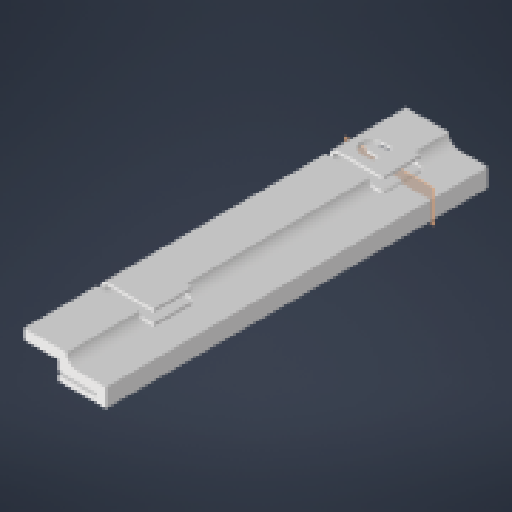
# Autodesk Inventor part: Tourniquet_Rail_01
Saved by Autodesk Inventor 2026.2 (Build 302298000, 298)
## iProperties
Created: 2026-03-04
Part Number: Tourniquet_Rail_01
Material: Generic
Document SubType Name: Modeling
Designer: vckot
Density: 1 g/cm^3
Appearance: Default
Author: vckot
Autodesk Inventor part; units mm, degrees
ref_plane "YZ Plane" through (0, 0, 0) normal (1, 0, 0) x (0, 1, 0)
ref_plane "XZ Plane" through (0, 0, 0) normal (0, 1, 0) x (-1, 0, 0)
ref_plane "XY Plane" through (0, 0, 0) normal (0, 0, 1) x (1, 0, 0)
sketch "Sketch1" plane through (0, 0, 0) normal (0, 1, 0) x (-1, 0, 0)
  line L0 (-6.25, 50) -> (6.25, 50)
  line L1 (6.25, 50) -> (6.25, -50)
  line L2 (6.25, -50) -> (-6.25, -50)
  line L3 (-6.25, -50) -> (-6.25, 50)
  line L4 (-6.25, 50) -> (6.25, -50) construction
  line L5 (6.25, 50) -> (-6.25, -50) construction
  point P0 (0, 0)
  dimension "d0" = 12.5
  dimension "d1" = 100
  constraints: 12 end point, 2 midpoint, 2 parallel, 1 horizontal, 1 perpendicular
  measures "d0" distance of L1.end L2.end
  measures "d1" distance of L0.end L1.end
extrude "Extrusion1" add sketch "Sketch1" along normal blind 4.8
sketch "Sketch2" plane through (-6.25, 0, -50) normal (-1, 0, 0) x (0, 0, 1)
  line L0 (0, 0) -> (0, 4.8) projected
  line L1 (100, 0) -> (100, 4.8) projected
  line L2 (0, 2.3) -> (100, 2.3)
  line L3 (100, 2.3) -> (100, 1.45)
  line L4 (100, 1.45) -> (0, 1.45)
  line L5 (0, 1.45) -> (0, 2.3)
  line L6 (0, 4.8) -> (100, 4.8) projected
  point P0 (50, 0)
  point P1 (100, 2.4)
  point P2 (0, 1.45)
  dimension "d4" = 0.85
  dimension "d7" = 2.5
  constraints: 8 end point, 2 parallel, 2 point on line, 1 horizontal, 1 midpoint, 1 perpendicular
  measures "d4" distance between parallel lines of L4 L2
  measures "d7" distance between parallel lines of L6 L2
extrude "Extrusion2" cut sketch "Sketch2" against normal blind 10 contours L0 L2 L1 L4
sketch "Sketch3" plane through (0, 4.8, 0) normal (0, 1, 0) x (1, 0, 0)
  line L0 (-6.25, 50) -> (-6.25, -50) projected
  line L1 (-6.25, -50) -> (-15.25, -50)
  line L2 (-15.25, -50) -> (-15.25, 50)
  line L3 (-15.25, 50) -> (-6.25, 50)
  line L4 (-6.25, 50) -> (-6.25, -50)
  line L5 (6.25, 50) -> (-6.25, 50) projected
  line L6 (-6.25, -50) -> (6.25, -50) projected
  line L7 (-6.25, 50) -> (-1.25, 50)
  line L8 (-1.25, 50) -> (-1.25, -50)
  line L9 (-1.25, -50) -> (-6.25, -50)
  line L10 (-6.25, -50) -> (-6.25, 50)
  point P0 (0, 0)
  dimension "d8" = 9
  dimension "d9" = 5
  constraints: 16 end point, 4 parallel, 2 horizontal, 2 perpendicular, 1 collinear, 1 point on line
  measures "d8" distance of L2.end L3.end
  measures "d9" distance of L8.end L9.end
extrude "Extrusion3" add sketch "Sketch3" along normal blind 2.75
fillet "Fillet1" radius 2.75 1 edges at (-1.25, 7.55, 0) inverted yes
sketch "Sketch4" plane through (6.25, 0, 50) normal (1, 0, 0) x (0, 0, -1)
  line L0 (100, 4.8) -> (0, 4.8) projected
  line L1 (100, 7.55) -> (0, 7.55) projected
  line L2 (79, 4.8) -> (91, 4.8)
  line L3 (91, 4.8) -> (91, 7.55)
  line L4 (91, 7.55) -> (79, 7.55)
  line L5 (79, 7.55) -> (79, 4.8)
  line L6 (0, 0) -> (0, 4.8) projected
  point P0 (50, 0)
  point P1 (85, 4.8)
  dimension "d13" = 85
  dimension "d14" = 12
  constraints: 8 end point, 2 parallel, 2 point on line, 1 horizontal, 1 midpoint, 1 perpendicular
  measures "d13" distance from line of L6 point (85, 4.8)
  measures "d14" distance between parallel lines of L3 L5
extrude "Extrusion4" cut sketch "Sketch4" against normal through all
ref_plane "Work Plane1" through (-6.25, 0, -35) normal (0, 0, 1) x (1, 0, 0)
sketch "Sketch5" plane through (-6.25, 0, -35) normal (0, 0, 1) x (1, 0, 0)
  arc A0 (-7, 8.8) -> (-7, 4.8) centre (-7, 6.8) ccw
  line L0 (-7, 4.8) -> (5, 4.8)
  line L1 (5, 4.8) -> (12.5, 4.8) projected
  line L2 (-9, 4.8) -> (0, 4.8) projected
  line L3 (-7, 8.8) -> (5, 8.8)
  line L4 (0, 2.3) -> (0, 4.8) projected
  line L5 (5, 8.05) -> (-7, 8.05)
  arc A1 (-7, 8.05) -> (-7, 5.55) centre (-7, 6.8) ccw
  line L6 (-7, 5.55) -> (5, 5.55)
  line L7 (5, 8.8) -> (5, 8.05)
  line L8 (5, 5.55) -> (5, 4.8)
  point P0 (6.25, 0)
  point P1 (-9, 6.8)
  dimension "d18" = 4
  dimension "d19" = 9
  dimension "d20" = 0.75
  constraints: 12 end point, 5 point on circle, 3 collinear, 2 centre point, 2 tangent, 1 horizontal, 1 horizontal alignment, 1 point on line, 1 vertical, 2 other
  measures "d18" diameter of A0
  measures "d19" distance from line of L4 point (-9, 6.8)
  measures "d20" distance between parallel lines of L3 L5
extrude "Extrusion5" add sketch "Sketch5" along normal mid plane 10
fillet "Fillet2" radius 0.75 1 edges at (-1.25, 5.55, -35)
sketch "Sketch6" plane through (-13.25, 8.8, -30) normal (0, 1, 0) x (1, 0, 0)
  line L0 (7, 4) -> (7, 2.5) projected
  line L1 (7, 2.5) -> (4, 2.5) projected
  line L2 (4, 7.5) -> (7, 7.5) projected
  line L3 (7, 7.5) -> (7, 6) projected
  line L4 (7, 6) -> (4, 6) projected
  arc A0 (4, 6) -> (4, 4) centre (4, 5) ccw projected
  line L5 (4, 4) -> (7, 4) projected
  line L6 (7, 4) -> (7, 2.5) projected
  line L7 (7, 2.5) -> (4, 2.5) projected
  arc A1 (4, 7.5) -> (4, 2.5) centre (4, 5) ccw projected
  arc A2 (4, 7.7) -> (4, 2.3) centre (4, 5) ccw
  line L8 (4, 7.7) -> (7, 7.7)
  line L9 (7, 2.3) -> (4, 2.3)
  line L10 (7, 2.3) -> (7, 2.5)
  line L11 (7, 7.7) -> (7, 7.5)
  point P0 (13.25, -30)
  point P1 (4, 2.3)
  dimension "d26" = 0.2
  dimension "d27" = 0.2
  dimension "d28" = 0.2
  constraints: 8 end point, 2 equal length, 2 point on circle, 1 centre point, 1 point on line, 1 vertical
  measures "d26" radial gap between concentric circles of A1 A2
  measures "d27" distance between parallel lines of L1 L9
  measures "d28" distance between parallel lines of L8 L2
extrude "Extrusion6" cut sketch "Sketch6" against normal blind 1
pattern_linear "Rectangular Pattern1" count 2 spacing 60 along (0, 0, 1) of "Extrusion5", "Extrusion4"
sketch "Sketch7" plane through (0, 4.8, 0) normal (0, 1, 0) x (1, 0, 0)
  circle A0 centre (0, -45) radius 1
  line L0 (-1.25, -50) -> (6.25, -50) projected
  line L1 (6.25, -50) -> (6.25, 50) projected
  circle A1 centre (0, -37.5) radius 1
  circle A2 centre (0, -30) radius 1
  circle A3 centre (0, -22.5) radius 1
  circle A4 centre (0, -15) radius 1
  circle A5 centre (0, -7.5) radius 1
  circle A6 centre (0, 0) radius 1
  circle A7 centre (0, 7.5) radius 1
  circle A8 centre (0, 15) radius 1
  circle A9 centre (0, 22.5) radius 1
  circle A10 centre (0, 30) radius 1
  circle A11 centre (0, 37.5) radius 1
  circle A12 centre (0, 45) radius 1
  point P0 (0, 0)
  dimension "d32" = 2
  dimension "d33" = 5
  dimension "d34" = 6.25
  dimension "d37" = 7.5
  constraints: 13 centre point, 1 vertical, 24 other
  measures "d32" diameter of A0
  measures "d33" distance from line of L0 A0.centre
  measures "d34" distance from line of L1 A0.centre
  measures "d37" distance of A0.centre A1.centre
extrude "Extrusion7" cut sketch "Sketch7" against normal through all
body "Solid1"
